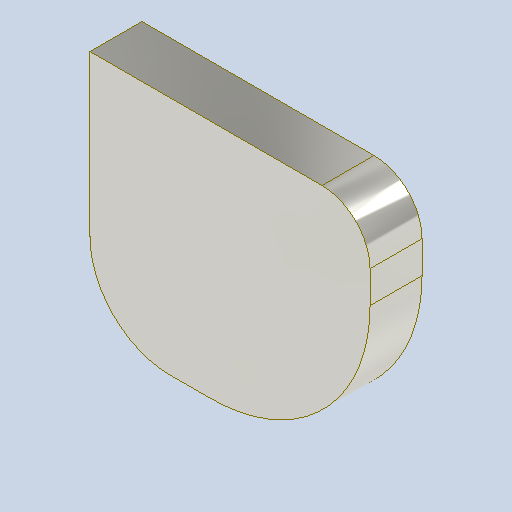
# Autodesk Inventor part: McCrea_oko_walle
Saved by Autodesk Inventor 2022 (Build 260153000, 153)
## iProperties
Created: 2022-01-17
Part Number: McCrea_oko_walle
Material: Generic
Document SubType Name: Modeling
Designer: student
Density: 1 g/cm^3
Appearance: Silver
Author: student
Autodesk Inventor part; units mm, degrees
ref_plane "YZ Plane" through (0, 0, 0) normal (1, 0, 0) x (0, 1, 0)
ref_plane "XZ Plane" through (0, 0, 0) normal (0, 1, 0) x (-1, 0, 0)
ref_plane "XY Plane" through (0, 0, 0) normal (0, 0, 1) x (1, 0, 0)
sketch "Sketch1" plane through (0, 0, 0) normal (0, 0, 1) x (1, 0, 0)
  line L0 (-11.9516, 53) -> (17.0484, 53)
  line L1 (23.0484, 47) -> (23.0484, 43)
  line L2 (3.0484, 23) -> (-1.9516, 23)
  line L3 (-11.9516, 33) -> (-11.9516, 53)
  arc A0 (23.0484, 47) -> (17.0484, 53) centre (17.0484, 47) ccw
  arc A1 (3.0484, 23) -> (23.0484, 43) centre (3.0484, 43) ccw
  arc A2 (-11.9516, 33) -> (-1.9516, 23) centre (-1.9516, 33) ccw
  point P0 (0, 0)
  point P1 (23.0484, 23)
  point P2 (-11.9516, 23)
  dimension "d0" = 6
  dimension "d1" = 30
  dimension "d2" = 35
  dimension "d3" = 20
  dimension "d4" = 10
  constraints: 8 end point, 6 point on circle, 6 tangent, 4 point on line, 3 centre point, 2 parallel, 1 horizontal, 1 perpendicular
  measures "d0" radius of A0
  measures "d1" distance of point (-11.952, 23) L0.start
  measures "d2" distance of point (23.048, 23) point (-11.952, 23)
  measures "d3" radius of A1
  measures "d4" radius of A2
extrude "Extrusion1" add sketch "Sketch1" along normal blind 5
sketch "Sketch3" plane through (0, 0, 0) normal (0, 0, -1) x (-1, 0, 0)
  line L0 (-17.0484, 53) -> (11.9516, 53) projected
  line L1 (11.9516, 53) -> (11.9516, 33) projected
  line L2 (11.9516, 53) -> (11.9516, 33)
  arc A0 (1.9516, 23) -> (11.9516, 33) centre (1.9516, 33) ccw projected
  line L3 (1.9516, 23) -> (-3.0484, 23) projected
  line L4 (1.9516, 23) -> (-3.0484, 23)
  line L5 (-23.0484, 43) -> (-23.0484, 47) projected
  line L6 (-23.0484, 43) -> (-23.0484, 47)
  arc A1 (-17.0484, 53) -> (-23.0484, 47) centre (-17.0484, 47) ccw projected
  line L7 (-17.0484, 53) -> (11.9516, 53)
  arc A2 (1.9516, 23) -> (11.9516, 33) centre (1.9516, 33) ccw
  arc A3 (-23.0484, 43) -> (-3.0484, 23) centre (-3.0484, 43) ccw
  arc A4 (-17.0484, 53) -> (-23.0484, 47) centre (-17.0484, 47) ccw
  line L8 (11.4516, 52.5) -> (11.4516, 33.5)
  line L9 (-2.5484, 23.5) -> (1.4516, 23.5)
  line L10 (-22.5484, 46.5) -> (-22.5484, 43.5)
  line L11 (-16.5484, 52.5) -> (11.4516, 52.5)
  arc A5 (-16.5484, 52.5) -> (-22.5484, 46.5) centre (-16.5484, 46.5) ccw
  arc A6 (1.4516, 23.5) -> (11.4516, 33.5) centre (1.4516, 33.5) ccw
  arc A7 (-22.5484, 43.5) -> (-2.5484, 23.5) centre (-2.5484, 43.5) ccw
  point P0 (0, 0)
  dimension "d14" = 10
  dimension "d15" = 20
  dimension "d16" = 6
  dimension "d17" = 0.5
  dimension "d18" = 0.5
  dimension "d19" = 0.5
  dimension "d20" = 0.5
  dimension "d21" = 6
  dimension "d22" = 10
  dimension "d23" = 20
  constraints: 16 end point, 13 tangent, 12 point on circle, 6 centre point, 6 point on line, 3 collinear, 1 horizontal, 1 parallel, 1 perpendicular, 1 vertical
  measures "d14" radius of A2
  measures "d15" radius of A3
  measures "d16" radius of A4
  measures "d17" distance between parallel lines of L0 L11
  measures "d18" distance between parallel lines of L1 L8
  measures "d19" distance between parallel lines of L3 L9
  measures "d20" distance between parallel lines of L6 L10
  measures "d21" radius of A5
  measures "d22" radius of A6
  measures "d23" radius of A7
extrude "Extrusion2" add sketch "Sketch3" along normal blind 1.5
body "Solid1"
